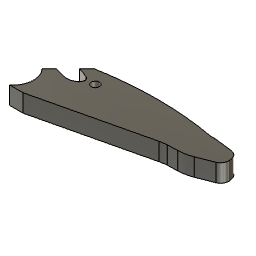
Finger1Section3P2V1 v2 (Autodesk Fusion 360 design; units mm, degrees)
Autodesk Fusion 360 part; units mm, degrees
sketch "Sketch1" plane through (0, 0, 0) normal (0, 0, 1) x (1, 0, 0)
  line L0 (4.6171, 4.1101) -> (5.507, 5)
  line L1 (20, 5) -> (20.5594, 5)
  line L2 (2.2748, 1.7678) -> (3.1661, 2.6591)
  arc A0 (19.5247, 1.403) -> (18.2667, 1.356) centre (20.507, -41.7412) ccw
  line L3 (2.007, -2) -> (3.6836, -2)
  line L4 (20.5594, 5) -> (22.8853, 4.7255)
  line L5 (37.507, -0.5557) -> (37.507, -2.0752)
  arc A1 (2.007, -2) -> (2.2748, 1.7678) centre (0.507, 0) ccw
  arc A2 (37.507, -0.5557) -> (33.9758, 3.4167) centre (33.507, -0.5557) ccw
  circle A3 centre (7.2949, 3.4) radius 0.5
  arc A4 (20, 5) -> (5.507, 5) centre (12.7535, -34.4243) ccw
  line L6 (3.6836, -2) -> (17.3695, 1.228)
  line L7 (23.8081, 3.6438) -> (23.7471, 3.9364)
  line L8 (23.1931, 2.5084) -> (21.248, 1.7482)
  arc A5 (23.7471, 3.9364) -> (22.8853, 4.7255) centre (22.7681, 3.7324) ccw
  arc A6 (23.1931, 2.5084) -> (23.8081, 3.6438) centre (22.8291, 3.4398) ccw
  arc A7 (19.5247, 1.403) -> (21.248, 1.7482) centre (19.4097, 6.4517) ccw
  arc A8 (18.2667, 1.356) -> (17.3695, 1.228) centre (18.5288, -3.6872) ccw
  line L9 (4.6171, 4.1101) -> (5.8592, 3.6736)
  line L10 (6.1934, 3.2018) -> (6.1934, 3.1451)
  line L11 (5.9851, 2.6906) -> (5.9361, 2.6483)
  line L12 (4.4874, 2.3121) -> (3.1644, 2.6574)
  arc A9 (6.1934, 3.2018) -> (5.8592, 3.6736) centre (5.6934, 3.2018) ccw
  arc A10 (5.9851, 2.6906) -> (6.1934, 3.1451) centre (5.5934, 3.1451) ccw
  arc A11 (4.4874, 2.3121) -> (5.9361, 2.6483) centre (4.8914, 3.8602) ccw
  dimension "d13" = 5
  dimension "d14" = 4
  dimension "d17" = 1
  dimension "d18" = 1.6
  dimension "d24" = 1
  dimension "d25" = 5.05
  dimension "d26" = 0.5
  dimension "d27" = 0.6
  dimension "d28" = 1.6
  constraint tangent L4 A2
  constraint tangent L5 A2
  constraint tangent L7 A5
  constraint tangent L4 A5
  constraint tangent L8 A6
  constraint tangent L7 A6
  constraint equal A5 A6
  constraint tangent L8 A7
  constraint tangent A0 A7
  constraint tangent A0 A8
  constraint tangent L6 A8
  constraint equal A7 A8
  constraint vertical L10
  constraint coincident L2 L12.end
  constraint tangent L9 A9
  constraint tangent L10 A9
  constraint tangent L10 A10
  constraint tangent L11 A10
  constraint tangent L11 A11
  constraint tangent L12 A11
  measures "d13" diameter of A1
  measures "d14" radius of A2
  measures "d17" diameter of A3
  measures "d18" distance of L1 A3.centre
  measures "d24" radius of A5
  measures "d25" radius of A7
  measures "d26" radius of A9
  measures "d27" radius of A10
  measures "d28" radius of A11
extrude "Extrude3" add sketch "Sketch1" along normal blind 2.2
